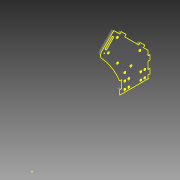
# Autodesk Inventor part: motor mount side
Saved by Autodesk Inventor 2015 (Build 190159000, 159)
## iProperties
Created: 2015-10-17
Part Number: motor mount side
Material: Polycarbonate, Clear
Document SubType Name: Modeling
Designer: Brian
Density: 1.2 g/cm^3
Appearance: Polycarbonate - Clear
Mass: 12.4998 g
Surface Area: 83.1912 cm^2
Volume: 10.4165 cm^3
Author: Brian
Autodesk Inventor part; units mm, degrees
ref_plane "YZ Plane" through (0, 0, 0) normal (1, 0, 0) x (0, 1, 0)
ref_plane "XZ Plane" through (0, 0, 0) normal (0, 1, 0) x (-1, 0, 0)
ref_plane "XY Plane" through (0, 0, 0) normal (0, 0, 1) x (1, 0, 0)
sketch "Sketch1" plane through (0, 0, 0) normal (1, 0, 0) x (0, 1, 0)
  line L0 (-51.6188, 88.6188) -> (0, 37) construction
  line L1 (0, 37) -> (0, 0) construction
  line L2 (0, 0) -> (-40, 0)
  line L3 (-40, 0) -> (-71.4178, 68.8198)
  line L4 (-51.6188, 88.6188) -> (-42.4264, 79.4264)
  line L5 (-40.3051, 81.5477) -> (-42.4264, 79.4264)
  line L6 (-40.3051, 81.5477) -> (-33.234, 74.4767)
  line L7 (-33.234, 74.4767) -> (-35.3553, 72.3553)
  line L8 (-35.3553, 72.3553) -> (-14.1421, 51.1421)
  line L9 (-14.1421, 51.1421) -> (-12.0208, 53.2635)
  line L10 (-12.0208, 53.2635) -> (-4.9497, 46.1924)
  line L11 (-4.9497, 46.1924) -> (-7.0711, 44.0711)
  line L12 (-7.0711, 44.0711) -> (0, 37)
  line L13 (0, 30) -> (3, 30)
  line L14 (3, 30) -> (3, 23)
  line L15 (3, 23) -> (0, 23)
  line L16 (0, 23) -> (0, 12)
  line L17 (0, 12) -> (3, 12)
  line L18 (3, 12) -> (3, 5)
  line L19 (3, 5) -> (0, 5)
  line L20 (0, 5) -> (0, 0)
  line L21 (0, 30) -> (0, 37)
  line L22 (-51.6188, 88.6188) -> (-71.4178, 68.8198)
  line L23 (-53.7401, 82.2548) -> (-51.6188, 80.1335)
  line L24 (-51.6188, 80.1335) -> (-62.9325, 68.8198)
  line L25 (-62.9325, 68.8198) -> (-65.0538, 70.9411)
  line L26 (-65.0538, 70.9411) -> (-53.7401, 82.2548)
  dimension "d3" = 40
  dimension "d5" = 135
  dimension "d6" = 28
  dimension "d10" = 73
  dimension "d11" = 37
  dimension "d14" = 10
  dimension "d15" = 10
  dimension "d16" = 10
  dimension "d17" = 7
  dimension "d18" = 5
  dimension "d19" = 7
  dimension "d20" = 7
  dimension "d21" = 3
  dimension "d25" = 6
  dimension "d26" = 6
  dimension "d27" = 3
  dimension "d28" = 3
  dimension "d29" = 13
  dimension "d30" = 3
  constraints: 55 end point, 12 perpendicular, 11 point on line, 3 collinear, 3 parallel, 1 coincident, 1 horizontal, 1 vertical
  measures "d3" distance of L1.end L2.end
  measures "d5" angle of L1 L0
  measures "d6" distance of L3.end L0.start
  measures "d10" distance of L0.start L0.end
  measures "d11" distance of L0.end L1.end
  measures "d14" distance of L5.start L6.end
  measures "d15" distance from line of L0.end L11
  measures "d16" distance of L9.end L10.end
  measures "d17" distance from line of L0.end L13
  measures "d18" vertical distance of point (0, 0) L18.end
  measures "d19" distance of L17.end L18.end
  measures "d20" distance of L13.end L14.end
  measures "d21" distance between parallel lines of L1 L18
  measures "d25" distance between parallel lines of L0 L23
  measures "d26" distance from line of L3.end L25
  measures "d27" distance between parallel lines of L22 L26
  measures "d28" distance of L24.end L25.end
  measures "d29" distance from line of L0.start L5
  measures "d30" distance between parallel lines of L0 L6
extrude "Extrusion1" add sketch "Sketch1" along normal blind 3
sketch "Sketch2" plane through (3, 0, 0) normal (1, 0, 0) x (0, 0, -1)
  circle A0 centre (-76.9515, -46.3155) radius 1.5
  line L0 (-76.9515, -46.3155) -> (-43.0104, -12.3744) construction
  line L1 (-43.0104, -12.3744) -> (-29.5754, -25.8094) construction
  line L2 (-29.5754, -25.8094) -> (-63.5165, -59.7505) construction
  line L3 (-63.5165, -59.7505) -> (-76.9515, -46.3155) construction
  line L4 (-51.1421, -14.1421) -> (-72.3553, -35.3553) construction
  line L5 (-80.1335, -51.6188) -> (-68.8198, -62.9325) construction
  circle A1 centre (-43.0104, -12.3744) radius 1.5
  circle A2 centre (-29.5754, -25.8094) radius 1.5
  circle A3 centre (-63.5165, -59.7505) radius 1.5
  point P0 (0, 0)
  dimension "d31" = 3
  dimension "d32" = 6
  dimension "d33" = 4.5
  dimension "d34" = 19
  dimension "d35" = 3
  dimension "d36" = 3
  dimension "d37" = 3
  dimension "d38" = 48
  constraints: 8 end point, 4 centre point, 3 coincident, 3 parallel, 1 perpendicular
  measures "d31" diameter of A0
  measures "d32" distance between parallel lines of L5 L3
  measures "d33" distance between parallel lines of L4 L0
  measures "d34" distance of L2.end L0.start
  measures "d35" diameter of A1
  measures "d36" diameter of A2
  measures "d37" diameter of A3
  measures "d38" distance of L1.end L2.end
extrude "Extrusion2" cut sketch "Sketch2" against normal blind 3
sketch "Sketch3" plane through (3, 0, 0) normal (1, 0, 0) x (0, 0, -1)
  circle A0 centre (-29.5754, -25.8094) radius 1.5 projected
  circle A1 centre (-76.9515, -46.3155) radius 1.5 projected
  circle A2 centre (-43.0104, -12.3744) radius 1.5 projected
  circle A3 centre (-63.5165, -59.7505) radius 1.5 projected
  line L0 (-80.1335, -51.6188) -> (-68.8198, -62.9325) projected
  line L1 (-68.8198, -62.9325) -> (-70.9411, -65.0538) projected
  line L2 (-70.9411, -65.0538) -> (-82.2548, -53.7401) projected
  line L3 (-82.2548, -53.7401) -> (-80.1335, -51.6188) projected
  line L4 (-79.4264, -42.4264) -> (-88.6188, -51.6188) projected
  line L5 (-88.6188, -51.6188) -> (-68.8198, -71.4178) projected
  line L6 (-68.8198, -71.4178) -> (0, -40) projected
  line L7 (0, -40) -> (0, 0) projected
  line L8 (0, 0) -> (-5, 0) projected
  line L9 (-5, 0) -> (-5, 3) projected
  line L10 (-5, 3) -> (-12, 3) projected
  line L11 (-12, 3) -> (-12, 0) projected
  line L12 (-12, 0) -> (-23, 0) projected
  line L13 (-23, 0) -> (-23, 3) projected
  line L14 (-23, 3) -> (-30, 3) projected
  line L15 (-30, 3) -> (-30, 0) projected
  line L16 (-30, 0) -> (-37, 0) projected
  line L17 (-37, 0) -> (-44.0711, -7.0711) projected
  line L18 (-44.0711, -7.0711) -> (-46.1924, -4.9497) projected
  line L19 (-46.1924, -4.9497) -> (-53.2635, -12.0208) projected
  line L20 (-53.2635, -12.0208) -> (-51.1421, -14.1421) projected
  line L21 (-51.1421, -14.1421) -> (-72.3553, -35.3553) projected
  line L22 (-72.3553, -35.3553) -> (-74.4767, -33.234) projected
  line L23 (-74.4767, -33.234) -> (-81.5477, -40.3051) projected
  line L24 (-81.5477, -40.3051) -> (-79.4264, -42.4264) projected
  arc A4 (0, -40) -> (-68.8198, -71.4178) centre (7.69, -147.9276) ccw
  line L25 (-68.8198, -71.4178) -> (-27.8142, -30.4121)
  line L26 (-51.1421, -14.1421) -> (-72.3553, -35.3553) projected
  constraints: 2 end point, 2 point on circle, 1 centre point, 1 parallel, 1 tangent
extrude "Extrusion3" cut sketch "Sketch3" against normal blind 3 contours A4 L6
sketch "Sketch4" plane through (3, 0, 0) normal (1, 0, 0) x (0, 0, -1)
  arc A0 (0, -40) -> (-68.8198, -71.4178) centre (7.69, -147.9276) ccw projected
  line L0 (0, -40) -> (0, 0) projected
  line L1 (0, 0) -> (-5, 0) projected
  line L2 (-5, 0) -> (-5, 3) projected
  line L3 (-5, 3) -> (-12, 3) projected
  line L4 (-12, 3) -> (-12, 0) projected
  line L5 (-12, 0) -> (-23, 0) projected
  line L6 (-23, 0) -> (-23, 3) projected
  line L7 (-23, 3) -> (-30, 3) projected
  line L8 (-30, 3) -> (-30, 0) projected
  line L9 (-30, 0) -> (-37, 0) projected
  line L10 (-37, 0) -> (-44.0711, -7.0711) projected
  line L11 (-44.0711, -7.0711) -> (-46.1924, -4.9497) projected
  line L12 (-46.1924, -4.9497) -> (-53.2635, -12.0208) projected
  line L13 (-53.2635, -12.0208) -> (-51.1421, -14.1421) projected
  line L14 (-51.1421, -14.1421) -> (-72.3553, -35.3553) projected
  line L15 (-72.3553, -35.3553) -> (-74.4767, -33.234) projected
  line L16 (-74.4767, -33.234) -> (-81.5477, -40.3051) projected
  line L17 (-81.5477, -40.3051) -> (-79.4264, -42.4264) projected
  line L18 (-79.4264, -42.4264) -> (-88.6188, -51.6188) projected
  line L19 (-88.6188, -51.6188) -> (-68.8198, -71.4178) projected
  circle A1 centre (-29.5754, -25.8094) radius 1.5 projected
  circle A2 centre (-76.9515, -46.3155) radius 1.5 projected
  circle A3 centre (-43.0104, -12.3744) radius 1.5 projected
  circle A4 centre (-63.5165, -59.7505) radius 1.5 projected
  line L20 (-80.1335, -51.6188) -> (-68.8198, -62.9325) projected
  line L21 (-68.8198, -62.9325) -> (-70.9411, -65.0538) projected
  line L22 (-70.9411, -65.0538) -> (-82.2548, -53.7401) projected
  line L23 (-82.2548, -53.7401) -> (-80.1335, -51.6188) projected
  line L24 (0, -40) -> (-18.724, -40)
  line L25 (-18.724, -43) -> (0, -43)
  line L26 (0, -43) -> (0, -40)
  line L27 (-18.724, -43) -> (-18.724, -40)
  dimension "d44" = 3
  constraints: 8 end point, 1 horizontal, 1 parallel, 1 perpendicular, 1 point on circle, 1 vertical
  measures "d44" distance of L25.end L0.start
extrude "Extrusion4" cut sketch "Sketch4" against normal blind 3 contours L26 L25 A0 | A0 L27 L24
sketch "Sketch5" plane through (3, 0, 0) normal (1, 0, 0) x (0, 0, -1)
  line L0 (-80.1335, -51.6188) -> (-68.8198, -62.9325) projected
  line L1 (-68.8198, -62.9325) -> (-70.9411, -65.0538) projected
  line L2 (-70.9411, -65.0538) -> (-82.2548, -53.7401) projected
  line L3 (-82.2548, -53.7401) -> (-80.1335, -51.6188) projected
  circle A0 centre (-63.5165, -59.7505) radius 1.5 projected
  circle A1 centre (-43.0104, -12.3744) radius 1.5 projected
  circle A2 centre (-76.9515, -46.3155) radius 1.5 projected
  circle A3 centre (-29.5754, -25.8094) radius 1.5 projected
  line L4 (-18.724, -43) -> (-18.724, -40) projected
  line L5 (-18.724, -40) -> (0, -40) projected
  line L6 (0, -40) -> (0, 0) projected
  line L7 (0, 0) -> (-5, 0) projected
  line L8 (-5, 0) -> (-5, 3) projected
  line L9 (-5, 3) -> (-12, 3) projected
  line L10 (-12, 3) -> (-12, 0) projected
  line L11 (-12, 0) -> (-23, 0) projected
  line L12 (-23, 0) -> (-23, 3) projected
  line L13 (-23, 3) -> (-30, 3) projected
  line L14 (-30, 3) -> (-30, 0) projected
  line L15 (-30, 0) -> (-37, 0) projected
  line L16 (-37, 0) -> (-44.0711, -7.0711) projected
  line L17 (-44.0711, -7.0711) -> (-46.1924, -4.9497) projected
  line L18 (-46.1924, -4.9497) -> (-53.2635, -12.0208) projected
  line L19 (-53.2635, -12.0208) -> (-51.1421, -14.1421) projected
  line L20 (-51.1421, -14.1421) -> (-72.3553, -35.3553) projected
  line L21 (-72.3553, -35.3553) -> (-74.4767, -33.234) projected
  line L22 (-74.4767, -33.234) -> (-81.5477, -40.3051) projected
  line L23 (-81.5477, -40.3051) -> (-79.4264, -42.4264) projected
  line L24 (-79.4264, -42.4264) -> (-88.6188, -51.6188) projected
  line L25 (-88.6188, -51.6188) -> (-68.8198, -71.4178) projected
  arc A4 (-18.724, -43) -> (-68.8198, -71.4178) centre (7.69, -147.9276) ccw projected
  line L26 (0, -40) -> (-18.724, -40) projected
  line L27 (0, -40) -> (-7, -40)
  line L28 (-7, -40) -> (-7, -43)
  line L29 (-7, -43) -> (0, -43)
  line L30 (0, -43) -> (0, -40)
  dimension "d47" = 3
  dimension "d48" = 7
  constraints: 8 end point, 2 parallel, 1 perpendicular, 1 point on line
  measures "d47" distance of L28.end L27.end
  measures "d48" distance of L28.end L29.end
extrude "Extrusion5" add sketch "Sketch5" against normal blind 3 contours L5 L30 L29 L28
sketch "Sketch6" plane through (3, 0, 0) normal (1, 0, 0) x (0, 0, -1)
  line L0 (-14.599, -5) -> (-3.599, -5) construction
  line L1 (-3.599, -5) -> (-3.599, -35) construction
  line L2 (-3.599, -35) -> (-14.599, -35) construction
  line L3 (-14.599, -35) -> (-14.599, -5) construction
  circle A0 centre (-3.599, -5) radius 1.5
  circle A1 centre (-14.599, -5) radius 1.5
  circle A2 centre (-14.599, -35) radius 1.5
  circle A3 centre (-14.599, -29) radius 1.5
  circle A4 centre (-14.599, -11) radius 1.5
  circle A5 centre (-3.599, -11) radius 1.5
  circle A6 centre (-3.599, -29) radius 1.5
  circle A7 centre (-3.599, -35) radius 1.5
  line L4 (0, 0) -> (0, -43) projected
  line L5 (-5, 0) -> (0, 0) projected
  line L6 (0, -43) -> (-7, -43) projected
  circle A8 centre (-25.599, -35) radius 1.5
  line L7 (-7, -43) -> (-7, -40) projected
  line L8 (-18.724, -40) -> (-18.724, -43) projected
  dimension "d51" = 3
  dimension "d52" = 3
  dimension "d53" = 3
  dimension "d54" = 3
  dimension "d55" = 3
  dimension "d56" = 3
  dimension "d57" = 3
  dimension "d58" = 3
  dimension "d59" = 3
  dimension "d62" = 3.599
  dimension "d63" = 5
  dimension "d64" = 11
  dimension "d65" = 6
  dimension "d66" = 6
  dimension "d67" = 5
  dimension "d68" = 11
  constraints: 9 centre point, 8 end point, 4 coincident, 4 point on line, 3 horizontal alignment, 2 parallel, 1 horizontal, 1 perpendicular
  measures "d51" diameter of A0
  measures "d52" diameter of A6
  measures "d53" diameter of A5
  measures "d54" diameter of A4
  measures "d55" diameter of A1
  measures "d56" diameter of A3
  measures "d57" diameter of A2
  measures "d58" diameter of A7
  measures "d59" diameter of A8
  measures "d62" distance between parallel lines of L4 L1
  measures "d63" distance between parallel lines of L5 L0
  measures "d64" distance of L0.start L0.end
  measures "d65" distance of L0.end A5.centre
  measures "d66" distance from line of L2 A6.centre
  measures "d67" distance from line of L7.end L2
  measures "d68" distance of L2.end A8.centre
extrude "Extrusion6" cut sketch "Sketch6" against normal blind 3
sketch "Sketch8" plane through (0, 0, 0) normal (-1, 0, 0) x (0, 0, 1)
  line L0 (68.8198, -71.4178) -> (48.209, -50.807)
  line L1 (48.209, -50.807) -> (45.3806, -53.6354)
  line L2 (45.3806, -53.6354) -> (65.9914, -74.2462)
  line L3 (65.9914, -74.2462) -> (68.8198, -71.4178)
  line L4 (88.6188, -51.6188) -> (68.8198, -71.4178) projected
  arc A0 (68.8198, -71.4178) -> (18.724, -43) centre (-7.69, -147.9276) ccw projected
  point P0 (0, 0)
  dimension "d70" = 4
  constraints: 8 end point, 2 parallel, 2 perpendicular, 1 point on circle
  measures "d70" distance of L2.end L0.start
extrude "Extrusion7" add sketch "Sketch8" against normal blind 3 contours L3 L2 A0
sketch "Sketch9" plane through (0, 0, 0) normal (-1, 0, 0) x (0, 0, 1)
  circle A0 centre (3.599, -35) radius 1.5 projected
  circle A1 centre (3.599, -11) radius 1.5 projected
  circle A2 centre (14.599, -29) radius 1.5 projected
  circle A3 centre (14.599, -5) radius 1.5 projected
  circle A4 centre (3.599, -5) radius 1.5 projected
  circle A5 centre (14.599, -35) radius 1.5 projected
  circle A6 centre (14.599, -11) radius 1.5 projected
  circle A7 centre (3.599, -29) radius 1.5 projected
  circle A8 centre (25.599, -35) radius 1.5 projected
  line L0 (18.724, -40) -> (18.724, -43) projected
  arc A9 (45.3806, -53.6354) -> (18.724, -43) centre (-7.69, -147.9276) ccw projected
  line L1 (45.3806, -53.6354) -> (65.9914, -74.2462) projected
  line L2 (65.9914, -74.2462) -> (88.6188, -51.6188) projected
  line L3 (88.6188, -51.6188) -> (79.4264, -42.4264) projected
  line L4 (79.4264, -42.4264) -> (81.5477, -40.3051) projected
  line L5 (81.5477, -40.3051) -> (74.4767, -33.234) projected
  line L6 (74.4767, -33.234) -> (72.3553, -35.3553) projected
  line L7 (72.3553, -35.3553) -> (51.1421, -14.1421) projected
  line L8 (51.1421, -14.1421) -> (53.2635, -12.0208) projected
  line L9 (53.2635, -12.0208) -> (46.1924, -4.9497) projected
  line L10 (46.1924, -4.9497) -> (44.0711, -7.0711) projected
  line L11 (44.0711, -7.0711) -> (37, 0) projected
  line L12 (37, 0) -> (30, 0) projected
  line L13 (30, 0) -> (30, 3) projected
  line L14 (30, 3) -> (23, 3) projected
  line L15 (23, 3) -> (23, 0) projected
  line L16 (23, 0) -> (12, 0) projected
  line L17 (12, 0) -> (12, 3) projected
  line L18 (12, 3) -> (5, 3) projected
  line L19 (5, 3) -> (5, 0) projected
  line L20 (5, 0) -> (0, 0) projected
  line L21 (0, 0) -> (0, -43) projected
  line L22 (0, -43) -> (7, -43) projected
  line L23 (7, -43) -> (7, -40) projected
  line L24 (7, -40) -> (18.724, -40) projected
  line L25 (68.8198, -62.9325) -> (80.1335, -51.6188) projected
  line L26 (80.1335, -51.6188) -> (82.2548, -53.7401) projected
  line L27 (82.2548, -53.7401) -> (70.9411, -65.0538) projected
  line L28 (70.9411, -65.0538) -> (68.8198, -62.9325) projected
  circle A10 centre (63.5165, -59.7505) radius 1.5 projected
  circle A11 centre (43.0104, -12.3744) radius 1.5 projected
  circle A12 centre (76.9515, -46.3155) radius 1.5 projected
  circle A13 centre (29.5754, -25.8094) radius 1.5 projected
  arc A14 (65.9914, -74.2462) -> (18.724, -43) centre (-34.2053, -174.4429) ccw
  constraints: 2 point on circle, 1 centre point, 1 tangent
extrude "Extrusion8" add sketch "Sketch9" against normal blind 3 contours A9 L1 A14
sketch "Sketch10" plane through (0, 0, 0) normal (-1, 0, 0) x (0, 0, 1)
  circle A0 centre (3.599, -35) radius 1.5 projected
  circle A1 centre (3.599, -11) radius 1.5 projected
  circle A2 centre (14.599, -29) radius 1.5 projected
  circle A3 centre (14.599, -5) radius 1.5 projected
  circle A4 centre (3.599, -5) radius 1.5 projected
  circle A5 centre (14.599, -35) radius 1.5 projected
  circle A6 centre (14.599, -11) radius 1.5 projected
  circle A7 centre (3.599, -29) radius 1.5 projected
  circle A8 centre (25.599, -35) radius 1.5 projected
  line L0 (18.724, -40) -> (18.724, -43) projected
  arc A9 (65.9914, -74.2462) -> (18.724, -43) centre (-34.2053, -174.4429) ccw projected
  line L1 (65.9914, -74.2462) -> (88.6188, -51.6188) projected
  line L2 (88.6188, -51.6188) -> (79.4264, -42.4264) projected
  line L3 (79.4264, -42.4264) -> (81.5477, -40.3051) projected
  line L4 (81.5477, -40.3051) -> (74.4767, -33.234) projected
  line L5 (74.4767, -33.234) -> (72.3553, -35.3553) projected
  line L6 (72.3553, -35.3553) -> (51.1421, -14.1421) projected
  line L7 (51.1421, -14.1421) -> (53.2635, -12.0208) projected
  line L8 (53.2635, -12.0208) -> (46.1924, -4.9497) projected
  line L9 (46.1924, -4.9497) -> (44.0711, -7.0711) projected
  line L10 (44.0711, -7.0711) -> (37, 0) projected
  line L11 (37, 0) -> (30, 0) projected
  line L12 (30, 0) -> (30, 3) projected
  line L13 (30, 3) -> (23, 3) projected
  line L14 (23, 3) -> (23, 0) projected
  line L15 (23, 0) -> (12, 0) projected
  line L16 (12, 0) -> (12, 3) projected
  line L17 (12, 3) -> (5, 3) projected
  line L18 (5, 3) -> (5, 0) projected
  line L19 (5, 0) -> (0, 0) projected
  line L20 (0, 0) -> (0, -43) projected
  line L21 (0, -43) -> (7, -43) projected
  line L22 (7, -43) -> (7, -40) projected
  line L23 (7, -40) -> (18.724, -40) projected
  line L24 (68.8198, -62.9325) -> (80.1335, -51.6188) projected
  line L25 (80.1335, -51.6188) -> (82.2548, -53.7401) projected
  line L26 (82.2548, -53.7401) -> (70.9411, -65.0538) projected
  line L27 (70.9411, -65.0538) -> (68.8198, -62.9325) projected
  circle A10 centre (63.5165, -59.7505) radius 1.5 projected
  circle A11 centre (43.0104, -12.3744) radius 1.5 projected
  circle A12 centre (76.9515, -46.3155) radius 1.5 projected
  circle A13 centre (29.5754, -25.8094) radius 1.5 projected
  circle A14 centre (43.364, -45.9619) radius 1.5
  dimension "d75" = 28
  dimension "d76" = 3
  dimension "d77" = 36
  constraints: 1 centre point
  measures "d75" distance from line of A14.centre L2
  measures "d76" diameter of A14
  measures "d77" distance from line of L1 A14.centre
extrude "Extrusion9" cut sketch "Sketch10" against normal blind 3 contours A14
fillet "Fillet2" radius 6 1 edges at (1.5, -74.2462, 65.9914)
sketch "Sketch11" plane through (3, 0, 0) normal (1, 0, 0) x (0, 0, -1)
  arc A0 (-70.1478, -70.0898) -> (-61.8384, -70.2586) centre (-65.9052, -65.8471) ccw projected
  arc A1 (-18.724, -43) -> (-61.8384, -70.2586) centre (34.2053, -174.4429) ccw projected
  line L0 (-18.724, -43) -> (-18.724, -40) projected
  line L1 (-18.724, -40) -> (-7, -40) projected
  line L2 (-7, -40) -> (-7, -43) projected
  line L3 (-7, -43) -> (0, -43) projected
  line L4 (0, -43) -> (0, 0) projected
  line L5 (0, 0) -> (-5, 0) projected
  line L6 (-5, 0) -> (-5, 3) projected
  line L7 (-5, 3) -> (-12, 3) projected
  line L8 (-12, 3) -> (-12, 0) projected
  line L9 (-12, 0) -> (-23, 0) projected
  line L10 (-23, 0) -> (-23, 3) projected
  line L11 (-23, 3) -> (-30, 3) projected
  line L12 (-30, 3) -> (-30, 0) projected
  line L13 (-30, 0) -> (-37, 0) projected
  line L14 (-37, 0) -> (-44.0711, -7.0711) projected
  line L15 (-44.0711, -7.0711) -> (-46.1924, -4.9497) projected
  line L16 (-46.1924, -4.9497) -> (-53.2635, -12.0208) projected
  line L17 (-53.2635, -12.0208) -> (-51.1421, -14.1421) projected
  line L18 (-51.1421, -14.1421) -> (-72.3553, -35.3553) projected
  line L19 (-72.3553, -35.3553) -> (-74.4767, -33.234) projected
  line L20 (-74.4767, -33.234) -> (-81.5477, -40.3051) projected
  line L21 (-81.5477, -40.3051) -> (-79.4264, -42.4264) projected
  line L22 (-79.4264, -42.4264) -> (-88.6188, -51.6188) projected
  line L23 (-88.6188, -51.6188) -> (-70.1478, -70.0898) projected
  circle A2 centre (-29.5754, -25.8094) radius 1.5 projected
  circle A3 centre (-76.9515, -46.3155) radius 1.5 projected
  circle A4 centre (-43.0104, -12.3744) radius 1.5 projected
  circle A5 centre (-63.5165, -59.7505) radius 1.5 projected
  line L24 (-80.1335, -51.6188) -> (-68.8198, -62.9325) projected
  line L25 (-68.8198, -62.9325) -> (-70.9411, -65.0538) projected
  line L26 (-70.9411, -65.0538) -> (-82.2548, -53.7401) projected
  line L27 (-82.2548, -53.7401) -> (-80.1335, -51.6188) projected
  circle A6 centre (-25.599, -35) radius 1.5 projected
  circle A7 centre (-3.599, -29) radius 1.5 projected
  circle A8 centre (-14.599, -11) radius 1.5 projected
  circle A9 centre (-14.599, -35) radius 1.5 projected
  circle A10 centre (-3.599, -5) radius 1.5 projected
  circle A11 centre (-14.599, -5) radius 1.5 projected
  circle A12 centre (-14.599, -29) radius 1.5 projected
  circle A13 centre (-3.599, -11) radius 1.5 projected
  circle A14 centre (-3.599, -35) radius 1.5 projected
  circle A15 centre (-43.364, -45.9619) radius 1.5 projected
equation "\"d21\" = d8"
equation "\"d26\" = d25"
equation "\"d30\" = d28"
equation "\"d35\" = d31"
equation "\"d36\" = d31"
equation "\"d37\" = d31"
equation "\"d52\" = d51"
equation "\"d53\" = d51"
equation "\"d54\" = d51"
equation "\"d55\" = d51"
equation "\"d56\" = d51"
equation "\"d57\" = d51"
equation "\"d58\" = d51"
equation "\"d59\" = d51"
equation "\"d67\" = d63"
equation "\"d8\" = 3"
body "Solid1"
